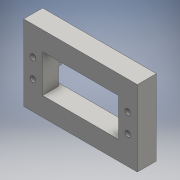
# Autodesk Inventor part: servoHolderTest1
Saved by Autodesk Inventor 2016 (Build 200138000, 138)
## iProperties
Created: 2016-04-16
Part Number: servoHolderTest1
Material: Generic
Document SubType Name: Modeling
Designer: hesaon
Density: 1 g/cm^3
Appearance: Default
Author: hesaon
Autodesk Inventor part; units mm, degrees
ref_plane "YZ Plane" through (0, 0, 0) normal (1, 0, 0) x (0, 1, 0)
ref_plane "XZ Plane" through (0, 0, 0) normal (0, 1, 0) x (-1, 0, 0)
ref_plane "XY Plane" through (0, 0, 0) normal (0, 0, 1) x (1, 0, 0)
sketch "Sketch1" plane through (0, 0, 0) normal (0, 1, 0) x (-1, 0, 0)
  line L0 (0, 0) -> (60, 0)
  line L1 (60, 0) -> (60, -40)
  line L2 (60, -40) -> (0, -40)
  line L3 (0, -40) -> (0, 0)
  line L4 (50, -10) -> (10, -10)
  line L5 (10, -10) -> (10, -30)
  line L6 (10, -30) -> (50, -30)
  line L7 (50, -30) -> (50, -10)
  circle A0 centre (55, -15) radius 1.5
  circle A1 centre (55, -25) radius 1.5
  circle A2 centre (5, -15) radius 1.5
  circle A3 centre (5, -25) radius 1.5
  dimension "d0" = 60
  dimension "d1" = 40
  dimension "d2" = 40
  dimension "d3" = 20
  dimension "d4" = 10
  dimension "d5" = 10
  dimension "d6" = 3
  dimension "d7" = 3
  dimension "d8" = 5
  dimension "d9" = 5
  dimension "d10" = 5
  dimension "d11" = 5
  dimension "d12" = 3
  dimension "d13" = 3
  dimension "d14" = 5
  dimension "d15" = 5
  dimension "d16" = 5
  dimension "d17" = 5
  constraints: 16 end point, 4 centre point, 4 parallel, 2 horizontal, 2 perpendicular
  measures "d0" distance of L1.end L2.end
  measures "d1" distance of L0.end L1.end
  measures "d2" distance of L4.end L4.start
  measures "d3" distance of L5.end L4.end
  measures "d4" distance from line of L3 L4.end
  measures "d5" distance from line of L0 L4.end
  measures "d6" diameter of A0
  measures "d7" diameter of A1
  measures "d8" distance from line of A0.centre L4
  measures "d9" distance from line of L7 A0.centre
  measures "d10" distance from line of L7 A1.centre
  measures "d11" distance from line of L6 A1.centre
  measures "d12" diameter of A2
  measures "d13" diameter of A3
  measures "d14" distance from line of L3 A3.centre
  measures "d15" distance from line of L6 A3.centre
  measures "d16" distance from line of L4 A2.centre
  measures "d17" distance from line of L3 A2.centre
extrude "Extrusion1" add sketch "Sketch1" along normal blind 10
sketch "Sketch2" plane through (0, 10, 0) normal (0, 1, 0) x (1, 0, 0)
  line L0 (-10, 30) -> (-2.5, 30)
  line L1 (-2.5, 30) -> (-2.5, 20.8)
  line L2 (-2.5, 20.8) -> (-10, 20.8)
  line L3 (-10, 20.8) -> (-10, 30)
  line L4 (-10, 10) -> (-2.5, 10)
  line L5 (-2.5, 10) -> (-2.5, 19.2)
  line L6 (-2.5, 19.2) -> (-10, 19.2)
  line L7 (-10, 19.2) -> (-10, 10)
  line L8 (0, 0) -> (0, 40) projected
  line L9 (-60, 0) -> (0, 0) projected
  line L10 (-57.5, 10) -> (-50, 10)
  line L11 (-50, 10) -> (-50, 19.2)
  line L12 (-50, 19.2) -> (-57.5, 19.2)
  line L13 (-57.5, 19.2) -> (-57.5, 10)
  line L14 (-57.5, 20.8) -> (-50, 20.8)
  line L15 (-50, 20.8) -> (-50, 30)
  line L16 (-50, 30) -> (-57.5, 30)
  line L17 (-57.5, 30) -> (-57.5, 20.8)
  line L18 (-60, 0) -> (-60, 40) projected
  dimension "d22" = 9.2
  dimension "d30" = 7.5
  dimension "d31" = 9.2
  dimension "d32" = 7.5
  dimension "d33" = 2.5
  dimension "d34" = 10
  dimension "d35" = 1.6
  dimension "d36" = 2.5
  dimension "d37" = 7.5
  dimension "d38" = 9.2
  dimension "d39" = 7.5
  dimension "d40" = 9.2
  dimension "d41" = 2.5
  dimension "d42" = 10
  dimension "d43" = 1.6
  dimension "d44" = 2.5
  constraints: 32 end point, 8 parallel, 4 horizontal, 4 perpendicular
  measures "d22" distance of L0.end L1.end
  measures "d30" distance of L0.end L0.start
  measures "d31" distance of L5.end L4.end
  measures "d32" distance of L4.end L4.start
  measures "d33" distance from line of L8 L4.end
  measures "d34" distance between parallel lines of L9 L4
  measures "d35" distance between parallel lines of L6 L2
  measures "d36" distance between parallel lines of L8 L1
  measures "d37" distance of L12.end L11.end
  measures "d38" distance of L11.end L10.end
  measures "d39" distance of L15.end L16.end
  measures "d40" distance of L16.end L14.start
  measures "d41" distance from line of L18 L10.start
  measures "d42" distance from line of L9 L10.start
  measures "d43" distance of L12.end L14.start
  measures "d44" distance from line of L18 L16.end
extrude "Extrusion2" cut sketch "Sketch2" against normal blind 1.6
body "Solid1"
